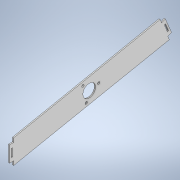
# Autodesk Inventor part: angularPlate
Saved by Autodesk Inventor 2020 (Build 240168000, 168)
## iProperties
Created: 2019-06-18
Part Number: angularPlate
Material: Generic
Document SubType Name: Modeling
Designer: Vivek Muskan
Density: 1 g/cm^3
Appearance: Default
Author: Vivek Muskan
Autodesk Inventor part; units mm, degrees
ref_plane "YZ Plane" through (0, 0, 0) normal (1, 0, 0) x (0, 1, 0)
ref_plane "XZ Plane" through (0, 0, 0) normal (0, 1, 0) x (-1, 0, 0)
ref_plane "XY Plane" through (0, 0, 0) normal (0, 0, 1) x (1, 0, 0)
sketch "Sketch3" plane through (0, 0, 0) normal (1, 0, 0) x (0, 1, 0)
  line L0 (39.6156, -196.5769) -> (39.0387, -195.1923)
  line L1 (39.0387, -195.1923) -> (85.1925, -175.9614)
  line L2 (39.6156, -196.5769) -> (85.7694, -177.346)
  line L3 (85.7694, -177.346) -> (85.1925, -175.9614)
  line L4 (0, 1.5) -> (50, 1.5)
  line L5 (0, 0) -> (50, 0)
  line L6 (50, 0) -> (50, 1.5)
  line L7 (0, 0) -> (0, 1.5)
  line L8 (0, 0) -> (39.0387, -195.1923)
  line L9 (39.0387, -195.1923) -> (66.731, -183.6537)
  line L10 (0, 0) -> (30, 0)
  line L11 (52.8848, -189.423) -> (15, 0)
  line L12 (39.0387, -195.1923) -> (43.6541, -193.2692)
  line L13 (43.6541, -193.2692) -> (62.1156, -185.5768)
  line L14 (62.1156, -185.5768) -> (64.0387, -190.1922)
  line L15 (64.0387, -190.1922) -> (45.5772, -197.8845)
  line L16 (45.5772, -197.8845) -> (43.6541, -193.2692)
  line L17 (43.6541, -193.2692) -> (48.2694, -191.3461)
  line L18 (48.2694, -191.3461) -> (48.8464, -192.7307)
  line L19 (48.8464, -192.7307) -> (58.0771, -188.8845)
  line L20 (58.0771, -188.8845) -> (58.6541, -190.2691)
  line L21 (58.6541, -190.2691) -> (49.4233, -194.1153)
  line L22 (49.4233, -194.1153) -> (48.8464, -192.7307)
  line L23 (66.731, -183.6537) -> (30, 0)
  line L24 (19.5193, -97.5961) -> (48.3655, -91.8269)
  circle A0 centre (33.9424, -94.7115) radius 8
  line L25 (20, 3) -> (10, 3)
  line L26 (10, 3) -> (10, 1.5)
  line L27 (0, 1.5) -> (50, 1.5)
  line L28 (20, 1.5) -> (20, 3)
  line L29 (25, 0) -> (25, 5)
  line L30 (25, 5) -> (5, 5)
  line L31 (5, 5) -> (5, 0)
  line L32 (33.9424, -94.7115) -> (36.2958, -106.4785)
  circle A1 centre (36.2958, -106.4785) radius 1.5
  circle A2 centre (42.9562, -86.7899) radius 1.5
  circle A3 centre (22.5752, -90.8661) radius 1.5
  dimension "d26" = 30
  dimension "d27" = 5
  dimension "d28" = 20
  dimension "d29" = 5
  dimension "d30" = 5
  dimension "d31" = 10
  dimension "d32" = 1.5
  dimension "d33" = 16
  dimension "d34" = 12
  dimension "d35" = 3
  dimension "d38" = 360
  constraints: 66 end point, 10 point on line, 8 symmetric about line, 5 midpoint, 4 centre point, 4 parallel, 3 perpendicular, 1 coincident, 7 other
  measures "d26" distance of L0.end L9.end
  measures "d27" distance of L0.end L12.end
  measures "d28" distance of L12.end L13.end
  measures "d29" distance of L13.end L14.end
  measures "d30" distance of L12.end L17.end
  measures "d31" distance of L18.end L19.end
  measures "d32" distance of L19.end L20.end
  measures "d33" diameter of A0
  measures "d34" distance of L32.start L32.end
  measures "d35" diameter of A1
extrude "Extrusion3" add sketch "Sketch3" along normal blind 1.5 contours L8 L24 A0 L11 A1 L1 | L16 L1 L18 L2 | L2 L22 L21 L20 L14 L15 L16 | L8 L5 L11 A0 L24 | L18 L1 L14 L2 | L11 A1 A0 L24 L23 L1 | L31 L4 L29 L5 | L11 L5 L23 L24 A0 | L31 L30 L29 L4 L28 L25 L26
body "Solid2"
